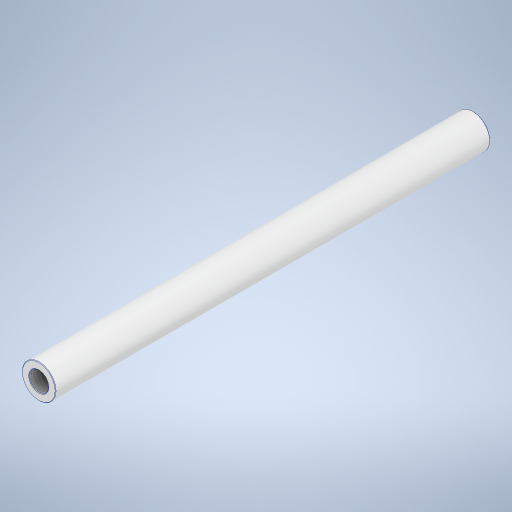
# Autodesk Inventor part: M4 85mm Standoff
Saved by Autodesk Inventor 2024 (Build 280153000, 153)
## iProperties
Created: 2024-12-26
Part Number: M4 85mm Standoff
Material: Aluminum 6061
Document SubType Name: Modeling
Designer: Ishaan
Density: 2.7 g/cm^3
Appearance: Aluminum - Flat
Author: Ishaan
Autodesk Inventor part; units mm, degrees
ref_plane "YZ Plane" through (0, 0, 0) normal (1, 0, 0) x (0, 1, 0)
ref_plane "XZ Plane" through (0, 0, 0) normal (0, 1, 0) x (-1, 0, 0)
ref_plane "XY Plane" through (0, 0, 0) normal (0, 0, 1) x (1, 0, 0)
sketch "Sketch1" plane through (0, 0, 0) normal (0, 0, 1) x (1, 0, 0)
  circle A0 centre (0, 0) radius 3.5
  circle A1 centre (0, 0) radius 2
  dimension "d0" = 7
  dimension "d1" = 4
  constraints: 2 centre point, 2 coincident
  measures "d0" diameter of A0
  measures "d1" diameter of A1
extrude "Extrusion1" add sketch "Sketch1" along normal mid plane 90
thread "Thread1" size "M4x0.7" class "6H" standard "ANSI Metric M Profile" length 10
thread "Thread2" size "M4x0.7" class "6H" standard "ANSI Metric M Profile" length 10
chamfer "Chamfer1" distance 0.1 angle 45 4 edges at (-3.5, 0, 45) (-2, 0, 45) (-2, 0, -45) (-3.5, 0, -45)
body "Solid1"
